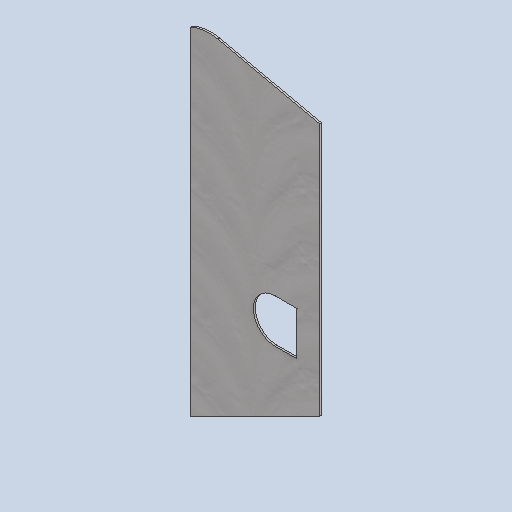
# Autodesk Inventor part: pokrywa prawa
Saved by Autodesk Inventor 2023 (Build 270158000, 158)
## iProperties
Created: 2022-10-11
Part Number: pokrywa prawa
Material: Stal miękka, spawana
Document SubType Name: Modeling
Designer: komputer
Density: 7.85 g/cm^3
Appearance: Spawane — stal miękka
Author: komputer
Autodesk Inventor part; units mm, degrees
ref_plane "YZ Plane" through (0, 0, 0) normal (1, 0, 0) x (0, 1, 0)
ref_plane "XZ Plane" through (0, 0, 0) normal (0, 1, 0) x (-1, 0, 0)
ref_plane "XY Plane" through (0, 0, 0) normal (0, 0, 1) x (1, 0, 0)
sketch "Sketch1" plane through (0, 0, 0) normal (0, 0, 1) x (1, 0, 0)
  line L0 (-17.5, -33.2499) -> (-17.5, 57.9837) projected
  arc A0 (-10.0449, 58.8745) -> (-17.5, 57.9837) centre (-12.5, 47.7794) ccw projected
  line L1 (-10.0449, 58.8745) -> (17.5, 52.7794) projected
  line L2 (17.5, 52.7794) -> (17.5, -15.7501) projected
  line L3 (17.5, -15.7501) -> (-17.5, -33.2499) projected
  line L4 (0.5, 7.1892) -> (0.5, 22.231) projected
  line L5 (0.5, 22.231) -> (-5.8925, 22.231) projected
  line L6 (-5.8925, 22.231) -> (-5.8925, 7.1892) projected
  line L7 (-5.8925, 7.1892) -> (0.5, 7.1892) projected
  point P0 (0, 0)
extrude "Extrusion1" add sketch "Sketch1" along normal blind 0.5 contours L0 A0 L1 L2 L3 | L7 L6 L5 L4
sketch "Sketch2" plane through (0, 0, 0.5) normal (0, 0, 1) x (1, 0, 0)
  line L0 (-1.5084, -24.1362) -> (-5.5333, -16.0863) projected
  line L1 (-5.5333, -16.0863) -> (-14.5107, -20.575) projected
  line L2 (-14.5107, -20.575) -> (-10.1014, -29.3938) projected
  arc A0 (-17.5, -30.0139) -> (-14.6056, -31.8027) centre (-15.5, -30.0139) ccw projected
  line L3 (-17.5, -30.0139) -> (-17.5, -1.8864) projected
  line L4 (-17.5, -1.8864) -> (-7.5, -1.8864) projected
  line L5 (-7.5, -1.8864) -> (-7.5, 7.5751) projected
  line L6 (-7.5, 7.5751) -> (-8.8, 7.5751) projected
  line L7 (-8.8, 26.3195) -> (-8.8, 7.5751) projected
  spline S0 degree 3 poles (-14.2046, 28.2052) (-13.4118, 28.2052) (-12.6544, 28.0226) (-10.9379, 27.4679) (-9.855, 26.8958) (-8.8077, 26.3237) (-8.8038, 26.3216) (-8.8, 26.3195) knots -0.001308 -0.001308 -0.001308 -0.001308 0.187612 0.187612 0.544343 0.544343 0.545651 0.545651 0.545651 0.545651 projected
  line L8 (-14.2046, 28.2052) -> (-17.5, 28.2052) projected
  line L9 (-17.5, 28.2052) -> (-17.5, 31.9794) projected
  arc A1 (-17.5, 31.9794) -> (-4.376, 33.2499) centre (-12.5, 48.7499) ccw projected
  arc A2 (-4.376, 33.2499) -> (2.7674, 54.4137) centre (-12.5, 47.7794) ccw projected
  arc A3 (3.9006, 55.7887) -> (2.7674, 54.4137) centre (3.6845, 54.8123) ccw projected
  line L10 (3.9006, 55.7887) -> (16.7161, 52.9529) projected
  arc A4 (17.5, 51.9765) -> (16.7161, 52.9529) centre (16.5, 51.9765) ccw projected
  line L11 (-17.5, 57.9837) -> (-17.5, -33.2499) projected
  line L12 (-17.5, -33.2499) -> (17.5, -15.7501) projected
  line L13 (17.5, -15.7501) -> (17.5, 52.7794) projected
  line L14 (17.5, 52.7794) -> (-10.0449, 58.8745) projected
  arc A5 (-10.0449, 58.8745) -> (-17.5, 57.9837) centre (-12.5, 47.7794) ccw projected
  line L15 (5.1606, 7.0459) -> (-1.321, 3.6769)
  line L16 (4.7678, -6.2957) -> (11.3303, -6.2957)
  line L17 (11.3303, -6.2957) -> (11.3303, 7.0459)
  circle A6 centre (5.4296, 0.5354) radius 5.9007
  line L18 (5.4296, 0.5354) -> (11.3303, 0.5354)
  line L19 (11.3303, 0.5354) -> (11.3303, 6.4362)
  line L20 (11.3303, 6.4362) -> (5.4296, 6.4362)
  line L21 (5.4296, 6.4362) -> (5.4296, 0.5354)
  line L22 (11.3303, 0.5354) -> (5.4296, 0.5354)
  line L23 (5.4296, 0.5354) -> (5.4296, -5.3653)
  line L24 (5.4296, -5.3653) -> (11.3303, -5.3653)
  line L25 (11.3303, -5.3653) -> (11.3303, 0.5354)
  line L26 (17.5, 51.9765) -> (17.5, -14.6321) projected
  line L27 (17.5, -14.6321) -> (-1.4167, -24.7491) projected
  arc A7 (-1.4167, -24.7491) -> (-1.5084, -24.1362) centre (-2.4029, -24.5834) ccw projected
  line L28 (-10.1014, -29.3938) -> (-14.6056, -31.8027) projected
  point P0 (0, 0)
  point P1 (17.5, 7.0459)
  point P2 (17.5, -15.0638)
  constraints: 22 end point, 4 parallel, 3 horizontal, 2 perpendicular, 2 point on line, 1 vertical, 4 other
extrude "Extrusion2" cut sketch "Sketch2" against normal blind 10 contours L24 A6 L17 | A6 L20 L17 | L18 L21 A6 | A6 L23 L18 | A6 L21 L23
body "Solid1"
